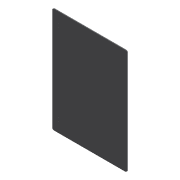
# Autodesk Inventor part: Standard
Saved by Autodesk Inventor 2020.3 (Build 243373000, 373)
## iProperties
RuleStatus: InUse
AfterDocSave0: file://Part Number Cleaner
Created: 2022-02-02
Material: Generic
Catalog Web Link: https://www.janelia.org/
Vendor: HHMI: JRC - jET
Document SubType Name: Modeling
Designer: solomone
Density: 1 g/cm^3
Appearance: Default
LAB/DEPT: A. LEE (LAB)
DESIGN DEPARTMENT: HHMI: JRC - jET
ALTERED ITEM PART NUMBER: N/A
ALTERED ITEM VENDOR: N/A
ALTERED ITEM DESCRIPTION: N/A
Title: Standard
Author: solomone
Revision Number: 0
Autodesk Inventor part; units mm, degrees
ref_plane "YZ Plane" through (0, 0, 0) normal (1, 0, 0) x (0, 1, 0)
ref_plane "XZ Plane" through (0, 0, 0) normal (0, 1, 0) x (-1, 0, 0)
ref_plane "XY Plane" through (0, 0, 0) normal (0, 0, 1) x (1, 0, 0)
sketch "Sketch1" plane through (0, 0, 0) normal (0, 0, 1) x (1, 0, 0)
  line L0 (-215.9, 304.8) -> (215.9, 304.8)
  line L1 (215.9, 304.8) -> (215.9, -304.8)
  line L2 (215.9, -304.8) -> (-215.9, -304.8)
  line L3 (-215.9, -304.8) -> (-215.9, 304.8)
  point P0 (0, 0)
  dimension "d0" = 431.8
  dimension "d1" = 609.6
  dimension "d2" = 304.8
  dimension "d3" = 215.9
  constraints: 8 end point, 2 parallel, 1 horizontal, 1 perpendicular
  measures "d0" distance of L0.start L0.end
  measures "d1" distance of L2.end L0.start
  measures "d2" distance from line of point (0, 0) L0
  measures "d3" distance from line of point (0, 0) L3
extrude "Extrusion1" add sketch "Sketch1" along normal blind 5
sketch "Sketch2" plane through (0, 0, 5) normal (0, 0, 1) x (1, 0, 0)
  line L0 (-215.9, -304.8) -> (215.9, -304.8) projected
  line L1 (-215.9, 304.8) -> (-215.9, -304.8) projected
  line L2 (215.9, 304.8) -> (-215.9, 304.8) projected
  line L3 (215.9, -304.8) -> (215.9, 304.8) projected
  point P0 (0, 0)
  point P1 (-179.25, -244)
  point P2 (-179.25, -224)
  point P3 (179.25, -244)
  point P4 (179.25, -224)
  point P5 (179.25, 224)
  point P6 (179.25, 244)
  point P7 (-179.25, 224)
  point P8 (-179.25, 244)
  point P9 (179.25, -117)
  point P10 (-179.25, -117)
  dimension "d6" = 20
  dimension "d7" = 60.8
  dimension "d8" = 36.65
  dimension "d16" = 20
  dimension "d17" = 60.8
  dimension "d18" = 36.65
  dimension "d20" = 127
  constraints: 8 vertical alignment, 5 horizontal alignment
  measures "d6" distance of point (-179.25, -224) point (-179.25, -244)
  measures "d7" distance from line of L0 point (-179.25, -244)
  measures "d8" distance from line of L1 point (-179.25, -244)
  measures "d16" distance of point (-179.25, 244) point (-179.25, 224)
  measures "d17" distance from line of L2 point (-179.25, 244)
  measures "d18" distance from line of L3 point (179.25, 244)
  measures "d20" distance of point (179.25, -117) point (179.25, -244)
hole "Hole1" at (-179.25, -244, 5) at (-179.25, -224, 5) at (-179.25, 224, 5) at (-179.25, 244, 5) at (179.25, 224, 5) at (179.25, 244, 5) at (179.25, -244, 5) at (179.25, -224, 5) at (179.25, -117, 5) at (-179.25, -117, 5) direction (0, 0, -1) diameter 3.4036 end through all clearance for "Flat Head Machine Screw" size "M3" standard "Ansi Metric M Profile"
fillet "Fillet1" radius 9.525 4 edges at (215.9, -304.8, 2.5) (-215.9, -304.8, 2.5) (215.9, 304.8, 2.5) (-215.9, 304.8, 2.5)
equation "\"d2\" = 0.5 * d1"
equation "\"d3\" = 0.5 * d0"
equation "\"d16\" = d6"
equation "\"d17\" = d7"
equation "\"d18\" = d8"
body "Solid1"
